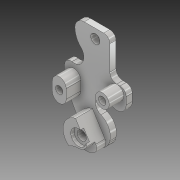
# Autodesk Inventor part: phalanx_2_housing_L
Saved by Autodesk Inventor 2017 SP1 (Build 210196100, 196)
## iProperties
Created: 2017-06-05
Part Number: phalanx_2_housing_L
Material: Generic
Document SubType Name: Modeling
Designer: Tomasz
Density: 1 g/cm^3
Appearance: Aluminum - Polished
Author: Tomasz
Autodesk Inventor part; units mm, degrees
ref_plane "YZ Plane" through (0, 0, 0) normal (1, 0, 0) x (0, 1, 0)
ref_plane "XZ Plane" through (0, 0, 0) normal (0, 1, 0) x (-1, 0, 0)
ref_plane "XY Plane" through (0, 0, 0) normal (0, 0, 1) x (1, 0, 0)
sketch "Sketch1" plane through (0, 0, 0) normal (0, 1, 0) x (-1, 0, 0)
  arc A0 (0, -5) -> (4.4, -2.3749) centre (0, 0) ccw
  line L0 (0, 0) -> (0, 30) construction
  line L1 (10, 9.2633) -> (10, 23)
  line L2 (5, 28) -> (0, 28)
  line L3 (9.4, 6.8883) -> (4.4, -2.3749)
  arc A1 (9.4, 6.8883) -> (10, 9.2633) centre (5, 9.2633) ccw
  arc A2 (-4.4, -2.3749) -> (0, -5) centre (0, 0) ccw
  line L4 (-10, 9.2633) -> (-10, 13.75)
  line L5 (-9.4, 6.8883) -> (-4.4, -2.3749)
  arc A3 (-10, 9.2633) -> (-9.4, 6.8883) centre (-5, 9.2633) ccw
  arc A4 (10, 23) -> (5, 28) centre (5, 23) ccw
  arc A5 (-6.95, 15.75) -> (-4.7, 18) centre (-6.95, 18) ccw
  line L6 (-6.95, 15.75) -> (-8, 15.75)
  line L7 (-4.7, 18) -> (-4.7, 26)
  line L8 (-2.7, 28) -> (0, 28)
  arc A6 (-2.7, 28) -> (-4.7, 26) centre (-2.7, 26) ccw
  arc A7 (-8, 15.75) -> (-10, 13.75) centre (-8, 13.75) ccw
  point P0 (10, 28)
  point P1 (10, 8)
  point P2 (-10, 15.75)
  point P3 (-4.7, 28)
  dimension "d0" = 10
  dimension "d3" = 10
  dimension "d4" = 28
  dimension "d26" = 8
  dimension "d27" = 5
  dimension "d47" = 5
  dimension "d81" = 3.05
  dimension "d82" = 2.25
  dimension "d83" = 10
  dimension "d84" = 2
  constraints: 18 end point, 16 point on circle, 11 tangent, 10 point on line, 8 centre point, 4 symmetric about line, 4 vertical, 2 coincident, 2 horizontal, 1 equal radius, 1 perpendicular, 2 other
  measures "d0" diameter of A0
  measures "d3" distance from line of L1 point (0, 0)
  measures "d4" distance from line of L2 point (0, 0)
  measures "d26" vertical distance of point (10, 8) point (0, 0)
  measures "d27" radius of A1
  measures "d47" radius of A4
  measures "d81" distance from line of A5.centre L4
  measures "d82" radius of A5
  measures "d83" distance from line of A5.centre L8
  measures "d84" radius of A6
extrude "Extrusion1" add sketch "Sketch1" along normal blind 2
sketch "Sketch3" plane through (0, 2, 0) normal (0, 1, 0) x (1, 0, 0)
  line L0 (0, 0) -> (0, -24.7147) construction
  line L1 (-5, -28) -> (2.7, -28) projected
  line L2 (-7, -8) -> (-7, -11) construction
  line L3 (-9.25, -8) -> (-9.25, -11)
  line L4 (-4.75, -11) -> (-4.75, -8)
  arc A0 (-4.75, -8) -> (-9.25, -8) centre (-7, -8) ccw
  arc A1 (-9.25, -11) -> (-4.75, -11) centre (-7, -11) ccw
  circle A2 centre (7, -13.5) radius 2.25
  point P0 (-10, -28)
  point P1 (10, -28)
  point P2 (5, -28)
  point P3 (2.254, -28)
  point P4 (4.7, -28)
  dimension "d28" = 14.5
  dimension "d29" = 7
  dimension "d70" = 7
  dimension "d71" = 20
  dimension "d173" = 4.5
  dimension "d174" = 3
  dimension "d175" = 4.5
  constraints: 10 end point, 4 point on circle, 4 tangent, 3 centre point, 2 vertical, 1 coincident, 1 parallel
  measures "d28" distance from line of point (7, -13.5) L1
  measures "d29" distance from line of point (7, -13.5) L0
  measures "d70" distance from line of L2.start L0
  measures "d71" distance from line of L2.start L1
  measures "d173" distance between parallel lines of L4 L3
  measures "d174" distance of L2.start L2.end
  measures "d175" diameter of A2
sketch "Sketch4" plane through (0, 0, 0) normal (0, -1, 0) x (1, 0, 0)
  line L0 (0, 0) -> (0, 33.5334) construction
  point P0 (0, 25)
  dimension "d37" = 25
  constraints: 2 end point, 1 point on line, 1 vertical
  measures "d37" distance of point (0, 25) L0.start
hole "Hole4" at (0, 0, 25) direction (0, 1, 0) diameter 3 end through all
sketch "Sketch5" plane through (0, 0, 0) normal (0, -1, 0) x (1, 0, 0)
  circle A0 centre (0, 0) radius 7.6158 construction
  line L0 (9.4, 6.8883) -> (4.4, -2.3749) projected
  arc A1 (7.4932, 1.3607) -> (2.7813, 7.0897) centre (0, 0) ccw construction
  line L1 (0, -0.8185) -> (0, 7.6158) construction
  arc A2 (7.613, -0.2064) -> (2.7813, 7.0897) centre (0, 0) ccw construction
  line L2 (4.4, -2.3749) -> (9.4, 6.8883) projected
  line L3 (0, 0) -> (12.3648, -3.6439) construction
  line L4 (0, 0) -> (4.576, 11.6645) construction
  arc A3 (3.7856, 9.6498) -> (1.777, 4.5297) centre (2.7813, 7.0897) ccw
  arc A4 (4.6673, -1.3754) -> (1.777, 4.5297) centre (0, 0) ccw
  arc A5 (8.7129, 5.6155) -> (3.7856, 9.6498) centre (0, 0) ccw
  line L5 (4.4, -2.3749) -> (4.6673, -1.3754)
  line L6 (8.7129, 5.6155) -> (4.4, -2.3749)
  dimension "d58" = 15.2316
  dimension "d63" = 21.42
  dimension "d64" = 5.5
  dimension "d65" = 85
  constraints: 12 point on circle, 10 end point, 6 centre point, 4 coincident, 4 point on line, 3 tangent, 2 concentric, 1 collinear, 1 vertical
  measures "d58" diameter of A0
  measures "d63" angle of L1 L4
  measures "d64" diameter of A3
  measures "d65" angle of L3 L4
extrude "Extrusion3" cut sketch "Sketch5" against normal through all
fillet "Fillet1" radius 3 1 edges at (4.4, 1, -2.3749)
fillet "Fillet2" radius 3 1 edges at (8.7129, 1, 5.6155)
sketch "Sketch6" plane through (0, 2, 0) normal (0, 1, 0) x (1, 0, 0)
  circle A0 centre (0, -25) radius 1.5 projected
  circle A1 centre (0, -25) radius 9.8995 construction
  line L0 (0, -25) -> (-14, -25) construction
  line L1 (0, -25) -> (-9.0301, -15.9194) construction
  arc A2 (-4.6888, -20.285) -> (-10, -16.7785) centre (-6.9804, -17.9805) ccw
  arc A3 (10, -11.3861) -> (5.4288, -8.8305) centre (7, -11.3861) ccw projected
  arc A4 (3.7856, -9.6498) -> (5.4288, -8.8305) centre (0, 0) ccw projected
  arc A5 (1.777, -4.5297) -> (3.7856, -9.6498) centre (2.7813, -7.0897) ccw projected
  arc A6 (1.777, -4.5297) -> (4.6673, 1.3754) centre (0, 0) ccw projected
  line L2 (-4.4, 2.3749) -> (-9.4, -6.8883) projected
  arc A7 (-9.4, -6.8883) -> (-10, -9.2633) centre (-5, -9.2633) ccw projected
  line L3 (-10, -9.2633) -> (-10, -23) projected
  arc A8 (-10, -23) -> (-5, -28) centre (-5, -23) ccw projected
  line L4 (-5, -28) -> (2.7, -28) projected
  line L5 (10, -13.75) -> (10, -11.3861) projected
  circle A9 centre (0, -25) radius 1.5 projected
  arc A10 (-4.6888, -20.285) -> (-5.9826, -27.9025) centre (0, -25) ccw
  line L6 (4.7, -26) -> (4.7, -18) projected
  arc A11 (6.95, -15.75) -> (4.7, -18) centre (6.95, -18) ccw projected
  line L7 (6.95, -15.75) -> (8, -15.75) projected
  arc A12 (2.7, -28) -> (4.7, -26) centre (2.7, -26) ccw projected
  arc A13 (8, -15.75) -> (10, -13.75) centre (8, -13.75) ccw projected
  arc A14 (4.5118, 1.9567) -> (4.0343, 2.9537) centre (1.6137, 1.1815) ccw projected
  line L8 (4.6673, 1.3754) -> (4.5118, 1.9567) projected
  arc A15 (4.0343, 2.9537) -> (-4.4, 2.3749) centre (0, 0) ccw projected
  dimension "d72" = 19.799
  dimension "d73" = 45.16
  dimension "d74" = 6.5
  constraints: 5 point on circle, 4 end point, 3 point on line, 2 centre point, 2 coincident, 1 horizontal, 3 other
  measures "d73" angle of L1 L0
  measures "d74" diameter of A2
extrude "Extrusion4" cut sketch "Sketch6" against normal through all contours A10 A8 L3 A2
fillet "Fillet3" radius 2 1 edges at (-10, 1, 16.7785)
fillet "Fillet4" radius 3 1 edges at (-5.9826, 1, 27.9025)
sketch "Sketch8" plane through (0, 0, 0) normal (0, -1, 0) x (1, 0, 0)
  arc A0 (4.0343, -2.9537) -> (4.5118, -1.9567) centre (1.6137, -1.1815) ccw projected
  arc A1 (4.6673, -1.3754) -> (1.777, 4.5297) centre (0, 0) ccw projected
  arc A2 (-3.6495, 28) -> (-6.6495, 25) centre (-3.6495, 25) ccw projected
  arc A3 (-6.6495, 25) -> (-4.6888, 20.285) centre (0, 25) ccw projected
  arc A4 (-7.6116, 14.7924) -> (-4.6888, 20.285) centre (-6.9804, 17.9805) ccw projected
  arc A5 (-7.6116, 14.7924) -> (-10, 12.8304) centre (-8, 12.8304) ccw projected
  line L0 (-10, 12.8304) -> (-10, 9.2633) projected
  arc A6 (-10, 9.2633) -> (-9.4, 6.8883) centre (-5, 9.2633) ccw projected
  line L1 (-9.4, 6.8883) -> (-4.4, -2.3749) projected
  arc A7 (4.6673, -1.3754) -> (1.777, 4.5297) centre (0, 0) ccw projected
  arc A8 (3.7856, 9.6498) -> (1.777, 4.5297) centre (2.7813, 7.0897) ccw projected
  arc A9 (5.4288, 8.8305) -> (3.7856, 9.6498) centre (0, 0) ccw projected
  arc A10 (5.4288, 8.8305) -> (10, 11.3861) centre (7, 11.3861) ccw projected
  line L2 (10, 11.3861) -> (10, 13.75) projected
  arc A11 (10, 13.75) -> (8, 15.75) centre (8, 13.75) ccw projected
  line L3 (8, 15.75) -> (6.95, 15.75) projected
  arc A12 (4.7, 18) -> (6.95, 15.75) centre (6.95, 18) ccw projected
  line L4 (4.7, 18) -> (4.7, 26) projected
  arc A13 (4.7, 26) -> (2.7, 28) centre (2.7, 26) ccw projected
  line L5 (2.7, 28) -> (-3.6495, 28) projected
  circle A14 centre (0, 25) radius 1.5 projected
  line L6 (-0.9453, 4.9096) -> (3.9983, -3.0019)
  line L7 (0, 0.4817) -> (0, -8.198)
  arc A15 (4.0343, -2.9537) -> (4.5118, -1.9567) centre (1.6137, -1.1815) ccw projected
  arc A16 (-4.4, -2.3749) -> (4.0343, -2.9537) centre (0, 0) ccw projected
  line L8 (4.5118, -1.9567) -> (4.6673, -1.3754) projected
  arc A17 (3.7856, 9.6498) -> (1.777, 4.5297) centre (2.7813, 7.0897) ccw projected
  arc A18 (-0.9453, 4.9096) -> (3.9983, -3.0019) centre (0, 0) ccw
  dimension "d90" = 32
  dimension "d97" = 1.8
  constraints: 4 end point, 2 point on circle, 1 centre point, 1 coincident, 1 point on line, 1 vertical, 2 other
  measures "d90" angle of L7 L6
  measures "d97" distance from line of point (0, 0) L6
extrude "Extrusion6" add sketch "Sketch8" along normal blind 5.5 contours A16 A18 L6
fillet "Fillet5" radius 2 1 edges at (3.9983, -2.75, -3.0019)
sketch "Sketch12" plane through (0, 2, 0) normal (0, 1, 0) x (1, 0, 0)
  line L0 (1.75, 3.0311) -> (3.5, 0) construction
  line L1 (3.5, 0) -> (1.75, -3.0311) construction
  line L2 (1.75, -3.0311) -> (-1.75, -3.0311) construction
  line L3 (-1.75, -3.0311) -> (-3.5, 0) construction
  line L4 (-3.5, 0) -> (-1.75, 3.0311) construction
  line L5 (-1.75, 3.0311) -> (1.75, 3.0311) construction
  line L6 (0, 0) -> (1.75, 3.0311) construction
  line L7 (0, 0) -> (0, 13.3212) construction
  dimension "d108" = 3.5
  dimension "d109" = 30
  constraints: 16 end point, 1 coincident, 1 vertical, 13 other
  measures "d108" distance of L6.start L0.start
  measures "d109" angle of L6 L7
sketch "Sketch19" plane through (0, -5.5, 0) normal (0, -1, 0) x (1, 0, 0)
  arc A0 (0, -3) -> (-3.1427, -3.8889) centre (0, -9) ccw
  arc A1 (3.8889, 3.1427) -> (3, 0) centre (9, 0) ccw
  arc A2 (0, -3) -> (3, 0) centre (0, 0) ccw
  arc A3 (-3.1427, -3.8889) -> (3.8889, 3.1427) centre (0, 0) ccw
  dimension "d148" = 12
  dimension "d149" = 12
  dimension "d150" = 9
  dimension "d151" = 9
  dimension "d152" = 10
  constraints: 8 point on circle, 4 centre point, 2 coincident, 1 horizontal alignment, 1 tangent, 1 vertical alignment
  measures "d148" diameter of A0
  measures "d149" diameter of A1
  measures "d150" distance of A1.centre point (0, 0)
  measures "d151" distance of A0.centre point (0, 0)
  measures "d152" diameter of A3
extrude "Extrusion8" cut sketch "Sketch19" against normal blind 2.5
sketch "Sketch20" plane through (0, 2, 0) normal (0, 1, 0) x (1, 0, 0)
  point P0 (0, 0)
  point P1 (0, 0)
  constraints: 1 coincident
hole "Hole10" at (0, 2, 0) direction (0, -1, 0) diameter 3 end through all
hole "Hole11" at (0, -5.5, 0) direction (0, 1, 0) diameter 5 depth 1.1
extrude "Extrusion9" add sketch "Sketch3" against normal blind 6.75
sketch "Sketch21" plane through (0, 2, 0) normal (0, 1, 0) x (1, 0, 0)
  arc A0 (-9.25, -11) -> (-4.75, -11) centre (-7, -11) ccw projected
  arc A1 (-4.75, -8) -> (-9.25, -8) centre (-7, -8) ccw projected
  line L0 (-7, -11) -> (-7, -8) construction
  circle A2 centre (7, -13.5) radius 2.25 projected
  point P0 (0, 0)
  point P1 (-7, -9.5)
  constraints: 2 end point, 1 coincident, 1 midpoint, 1 vertical
hole "Hole12" at (-7, 2, 9.5) at (7, 2, 13.5) direction (0, -1, 0) diameter 2.4 end through all countersink diameter 4.2 countersink angle 90
equation "\"d150\" = gear_distance_4_5"
equation "\"d151\" = gear_distance_4_5"
equation "\"gear_distance_4_5\" = 9"
body "Solid1"
